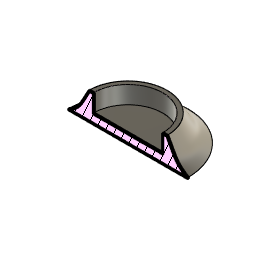
3D CNC Version 5 v8 (Autodesk Fusion 360 archive; units mm, degrees)
design "TestFitCandleHolder"
Autodesk Fusion 360 part; units mm, degrees
sketch "Sketch1" plane through (0, 0, 0) normal (0, 0, 1) x (1, 0, 0)
  circle A0 centre (0, 0) radius 19.75
  circle A1 centre (0, 0) radius 22.25
  dimension "d1" = 39.5
  dimension "d2" = 44.5
  constraint coincident A0.centre A1.centre
  measures "d1" diameter of A0
  measures "d2" diameter of A1
extrude "Extrude1" add sketch "Sketch1" along normal blind 5 contours A0
extrude "Extrude2" add sketch "Sketch1" along normal blind 15
sketch "Sketch2" plane through (0, 0, 0) normal (1, 0, 0) x (0, 1, 0)
  spline S0 degree 2 poles (-22.2, 15) (-28, 4) (-34, 0) knots 0 0 0 1.939246 1.939246 1.939246 weights 1 3 1
  line L0 (-22.2, 15) -> (-22.2, 0)
  line L1 (-22.2, 0) -> (-34, 0)
  constraint vertical L0
  constraint perpendicular L0 L1
revolve "Revolve1" add sketch "Sketch2" angle 360 about axis through (0, 0, 1.75) along (0, 0, 1)
